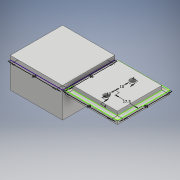
# Autodesk Inventor part: Camera_Display_Box
Saved by Autodesk Inventor 2017 (Build 210142000, 142)
## iProperties
Created: 2017-03-26
Part Number: Camera_Display_Box
Material: Generic
Document SubType Name: Modeling
Designer: willt
Density: 1 g/cm^3
Appearance: Default
Author: willt
Autodesk Inventor part; units mm, degrees
ref_plane "YZ Plane" through (0, 0, 0) normal (1, 0, 0) x (0, 1, 0)
ref_plane "XZ Plane" through (0, 0, 0) normal (0, 1, 0) x (-1, 0, 0)
ref_plane "XY Plane" through (0, 0, 0) normal (0, 0, 1) x (1, 0, 0)
sketch "Sketch1" plane through (0, 0, 0) normal (0, 0, 1) x (1, 0, 0)
  line L0 (-20, 20) -> (20, 20)
  line L1 (20, 20) -> (20, -20)
  line L2 (20, -20) -> (-20, -20)
  line L3 (-20, -20) -> (-20, 20)
  line L4 (-20, 20) -> (20, -20) construction
  line L5 (20, 20) -> (-20, -20) construction
  line L6 (-17, 17) -> (17, 17)
  line L7 (17, 17) -> (17, -17)
  line L8 (17, -17) -> (-17, -17)
  line L9 (-17, -17) -> (-17, 17)
  line L10 (-17, 17) -> (17, -17) construction
  line L11 (17, 17) -> (-17, -17) construction
  line L12 (20.9643, 21) -> (60.9643, 21)
  line L13 (60.9643, 21) -> (60.9643, -19)
  line L14 (60.9643, -19) -> (20.9643, -19)
  line L15 (20.9643, -19) -> (20.9643, 21)
  line L16 (20.9643, 21) -> (60.9643, -19) construction
  line L17 (60.9643, 21) -> (20.9643, -19) construction
  line L18 (23.9643, 18) -> (57.9643, 18)
  line L19 (57.9643, 18) -> (57.9643, -16)
  line L20 (57.9643, -16) -> (23.9643, -16)
  line L21 (23.9643, -16) -> (23.9643, 18)
  line L22 (23.9643, 18) -> (57.9643, -16) construction
  line L23 (57.9643, 18) -> (23.9643, -16) construction
  line L24 (60.9643, 0) -> (43.4643, 0) construction
  line L25 (43.4643, 0) -> (43.4643, -10) construction
  line L26 (43.4643, 0) -> (43.4643, 10) construction
  circle A0 centre (43.4643, -10) radius 2
  circle A1 centre (43.4643, 10) radius 2
  point P0 (0, 0)
  point P1 (40.9643, 1)
  dimension "d0" = 40
  dimension "d1" = 40
  dimension "d2" = 34
  dimension "d3" = 34
  dimension "d4" = 40
  dimension "d5" = 40
  dimension "d6" = 34
  dimension "d7" = 34
  dimension "d20" = 17.5
  dimension "d21" = 10
  dimension "d22" = 10
  dimension "d23" = 4
  dimension "d24" = 4
  constraints: 54 end point, 8 midpoint, 8 parallel, 5 horizontal, 5 perpendicular, 2 centre point, 2 coincident, 1 point on line, 1 vertical
  measures "d0" distance of L1.end L2.end
  measures "d1" distance of L0.end L1.end
  measures "d2" distance of L7.end L8.end
  measures "d3" distance of L6.end L7.end
  measures "d4" distance of L13.end L14.end
  measures "d5" distance of L12.end L13.end
  measures "d6" distance of L19.end L20.end
  measures "d7" distance of L18.end L19.end
  measures "d20" distance of L24.start L24.end
  measures "d21" distance of L24.end L25.end
  measures "d22" distance of L24.end L26.end
  measures "d23" diameter of A0
  measures "d24" diameter of A1
extrude "Extrusion7" add sketch "Sketch1" along normal blind 3 contours L0 L1 L2 L3 | L6 L7 L8 L9
extrude "Extrusion8" add sketch "Sketch1" against normal blind 20 contours L0 L1 L2 L3
extrude "Extrusion9" add sketch "Sketch1" along normal blind 3 contours L18 L19 L20 L21
extrude "Extrusion10" add sketch "Sketch1" against normal blind 3 contours L12 L13 L14 L15 | L18 L19 L20 L21
sketch "Sketch2" plane through (20, -20, 3) normal (1, 0, 0) x (0, 0, -1)
  line L0 (23, 0) -> (0, 0)
  line L1 (0, 0) -> (0, 40)
  line L2 (0, 40) -> (23, 40)
  line L3 (23, 40) -> (23, 0)
  point P0 (3, 20)
  constraints: 8 end point, 2 parallel, 1 horizontal, 1 perpendicular
split body "Split1" sketch "Sketch2" result two bodies curves L3 L0 L1 L2 first body at (34.2976, 20.5, -1)
body "Solid3"
body "Solid4"
